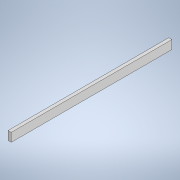
# Autodesk Inventor part: lw_6_part3
Saved by Autodesk Inventor 2021 (Build 250183000, 183)
## iProperties
Created: 2021-05-17
Part Number: lw_6_part3
Material: Типовые
Document SubType Name: Modeling
Designer: davam
Density: 1 g/cm^3
Appearance: По умолчанию
Author: davam
Autodesk Inventor part; units mm, degrees
ref_plane "YZ Plane" through (0, 0, 0) normal (1, 0, 0) x (0, 1, 0)
ref_plane "XZ Plane" through (0, 0, 0) normal (0, 1, 0) x (-1, 0, 0)
ref_plane "XY Plane" through (0, 0, 0) normal (0, 0, 1) x (1, 0, 0)
sketch "Эскиз1" plane through (0, 0, 0) normal (1, 0, 0) x (0, 1, 0)
  line L0 (8.3168, 848.3168) -> (-45.5446, 848.3168)
  line L1 (-45.5446, 848.3168) -> (-45.5446, -151.6832)
  line L2 (-45.5446, -151.6832) -> (8.3168, -151.6832)
  line L3 (8.3168, -151.6832) -> (8.3168, 848.3168)
  point P0 (0, 0)
  dimension "d0" = 1000
  constraints: 8 end point, 2 parallel, 1 horizontal, 1 perpendicular
  measures "d0" distance of L2.end L0.start
extrude "Выдавливание1" add sketch "Эскиз1" against normal blind 20
